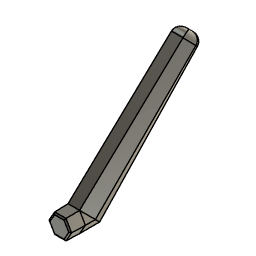
Drying_peg_10cm (Autodesk Fusion 360 design; units mm, degrees)
Autodesk Fusion 360 part; units mm, degrees
sketch "Sketch1" plane through (0, 0, 0) normal (0, 1, 0) x (1, 0, 0)
  line L0 (65, 37.5278) -> (0, 75.0555)
  line L1 (0, 75.0555) -> (-65, 37.5278)
  line L2 (-65, 37.5278) -> (-65, -37.5278)
  line L3 (-65, -37.5278) -> (0, -75.0555)
  line L4 (0, -75.0555) -> (65, -37.5278)
  line L5 (65, -37.5278) -> (65, 37.5278)
  line L6 (55, 31.7543) -> (0, 63.5085)
  line L7 (0, 63.5085) -> (-55, 31.7543)
  line L8 (-55, 31.7543) -> (-55, -31.7543)
  line L9 (-55, -31.7543) -> (0, -63.5085)
  line L10 (0, -63.5085) -> (55, -31.7543)
  line L11 (55, -31.7543) -> (55, 31.7543)
  dimension "d1" = 130
  dimension "d2" = 110
  measures "d1" distance of L2 L5
  measures "d2" distance of L8 L11
extrude "Extrude1" add sketch "Sketch1" against normal blind 7 contours L6 L7 L8 L9 L10 L11
ref_plane "WorkPlane3" through (0, 90, 0) normal (0, 1, 0) x (1, 0, 0)
sketch "Sketch3" plane through (0, 90, 0) normal (0, 1, 0) x (1, 0, 0)
  line L0 (-67, -38.6825) -> (0, -77.3649)
  line L1 (0, -77.3649) -> (67, -38.6825)
  line L2 (67, -38.6825) -> (67, 38.6825)
  line L3 (67, 38.6825) -> (0, 77.3649)
  line L4 (0, 77.3649) -> (-67, 38.6825)
  line L5 (-67, 38.6825) -> (-67, -38.6825)
  dimension "d9" = 134
  measures "d9" distance of L2 L5
loft "Loft1" add profiles "Sketch1", "Sketch3" section 1 section 2
loft "Loft2" add profiles "Sketch1" section 1 face at (0, -7, 0) section 2
sketch "Sketch4" plane through (0, 90, 0) normal (0, 1, 0) x (-1, 0, 0)
  line L0 (-67, 38.6825) -> (-67, -38.6825)
  line L1 (-67, -38.6825) -> (0, -77.3649)
  line L2 (0, -77.3649) -> (67, -38.6825)
  line L3 (67, -38.6825) -> (67, 38.6825)
  line L4 (67, 38.6825) -> (0, 77.3649)
  line L5 (0, 77.3649) -> (-67, 38.6825)
move_body "Move1" bodies 1 to x (0.866025, 0, 0.5) y (0, 1, 0) z (-0.5, 0, 0.866025) at (0, 0, 0)
ref_plane "WorkPlane4" through (0, 167, 0) normal (0, 1, 0) x (-0.5, 0, 0.866025)
extrude "Extrude2" add 1 faces at (-25.7883, 90, 0) along direction (0, 1, 0) blind 150
ref_plane "WorkPlane5" through (0, 90, 67) normal (0, 0.707107, 0.707107) x (1, 0, 0)
sketch "Sketch6" plane through (0, 78.5, 78.5) normal (0, 0.707107, 0.707107) x (1, 0, 0)
  line L0 (170, -150) -> (-170, -150)
  line L1 (-170, -150) -> (-170, 260)
  line L2 (-170, 260) -> (170, 260)
  line L3 (170, 260) -> (170, -150)
  constraint horizontal L0
  constraint vertical L1
  constraint horizontal L2
  constraint vertical L3
extrude "Extrude3" cut sketch "Sketch6" along normal blind 130
sketch "Sketch7" plane through (0, 78.5, 78.5) normal (0, 0.707107, 0.707107) x (-1, 0, 0)
  line L0 (38.6825, -16.2635) -> (-38.6825, -16.2635)
  line L1 (-38.6825, -16.2635) -> (-77.3649, -111.0158)
  line L2 (-77.3649, -111.0158) -> (-38.6825, -205.7681)
  line L3 (-38.6825, -205.7681) -> (38.6825, -205.7681)
  line L4 (38.6825, -205.7681) -> (77.3649, -111.0158)
  line L5 (77.3649, -111.0158) -> (38.6825, -16.2635)
ref_plane "WorkPlane6" through (0, 864.1068, 707.1068) normal (0, 0.707107, 0.707107) x (-1, 0, 0)
sketch "Sketch8" plane through (0, 785.6068, 785.6068) normal (0, 0.707107, 0.707107) x (-1, 0, 0)
  line L0 (-38.6825, -44.016) -> (-77.3649, -111.016)
  line L1 (-77.3649, -111.016) -> (-38.6825, -178.016)
  line L2 (-38.6825, -178.016) -> (38.6825, -178.016)
  line L3 (38.6825, -178.016) -> (77.3649, -111.016)
  line L4 (77.3649, -111.016) -> (38.6825, -44.016)
  line L5 (38.6825, -44.016) -> (-38.6825, -44.016)
  line L6 (38.6825, -16.2635) -> (-38.6825, -16.2635)
  line L7 (-38.6825, -205.7681) -> (38.6825, -205.7681)
  point P0 (0, -111.016)
  dimension "d18" = 134
  dimension "d19" = 27.7525
  dimension "d20" = 27.7521
  measures "d18" distance of L2 L5
  measures "d19" distance of L5 L6
  measures "d20" distance of L2 L7
loft "Loft3" add profiles "Sketch8", "Sketch7" section 1 section 2
fillet "Fillet1" radius 50 1 faces at (0, 864.1069, 707.1066)
